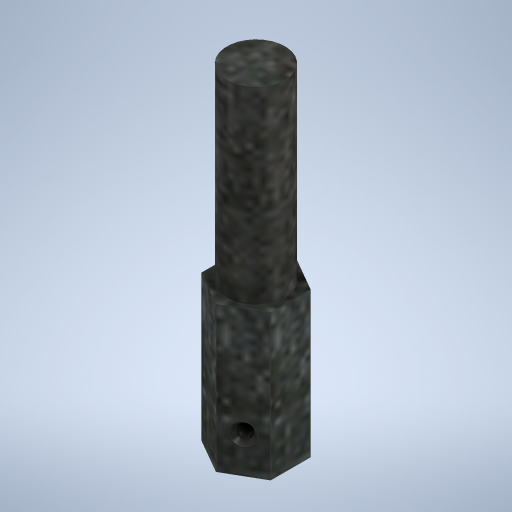
# Autodesk Inventor part: bevel gear shaft connector for versaball
Saved by Autodesk Inventor 2023 (Build 270158030, 158C)
## iProperties
Created: 2022-10-20
Part Number: bevel gear shaft connector for versaball
Material: Steel
Document SubType Name: Modeling
Designer: cjj5381
Density: 7.85 g/cm^3
Appearance: Plate
Author: cjj5381
Autodesk Inventor part; units mm, degrees
ref_plane "YZ Plane" through (0, 0, 0) normal (1, 0, 0) x (0, 1, 0)
ref_plane "XZ Plane" through (0, 0, 0) normal (0, 1, 0) x (-1, 0, 0)
ref_plane "XY Plane" through (0, 0, 0) normal (0, 0, 1) x (1, 0, 0)
sketch "Sketch1" plane through (0, 0, 0) normal (0, 1, 0) x (-1, 0, 0)
  line L0 (0, -5.4993) -> (-4.7625, -2.7496)
  line L1 (-4.7625, -2.7496) -> (-4.7625, 2.7496)
  line L2 (-4.7625, 2.7496) -> (0, 5.4993)
  line L3 (0, 5.4993) -> (4.7625, 2.7496)
  line L4 (4.7625, 2.7496) -> (4.7625, -2.7496)
  line L5 (4.7625, -2.7496) -> (0, -5.4993)
  point P0 (0, 0)
  point P1 (0, 0)
  dimension "d0" = 9.525
  constraints: 12 end point, 1 coincident, 13 other
  measures "d0" distance between parallel lines of L1 L4
extrude "Extrusion1" add sketch "Sketch1" along normal blind 20
sketch "Sketch2" plane through (0, 20, 0) normal (0, 1, 0) x (1, 0, 0)
  circle A0 centre (0, 0) radius 4
  dimension "d3" = 8
  constraints: 1 centre point, 1 coincident
  measures "d3" diameter of A0
extrude "Extrusion2" add sketch "Sketch2" along normal blind 5
sketch "Sketch4" plane through (4.7625, 0, 2.7496) normal (0.5, 0, 0.8660254) x (0.8660254, 0, -0.5)
  line L0 (-5.4993, 0) -> (0, 0) projected
  line L1 (0, 0) -> (0, 20) projected
  point P0 (-2.7496, 0)
  point P1 (-2.75, 5)
  dimension "d13" = 5
  dimension "d21" = 2.75
  measures "d13" distance from line of L0 point (-2.75, 5)
  measures "d21" distance from line of L1 point (-2.75, 5)
hole "Hole1" at (2.3809, 5, 4.1246) direction (-0.5, 0, -0.8660254) diameter 2 end through all countersink diameter 3 countersink angle 82
sketch "Sketch5" plane through (0, 25, 0) normal (0, 1, 0) x (1, 0, 0)
  circle A0 centre (0, 0) radius 4 projected
  circle A1 centre (0, 0) radius 4
  constraints: 1 centre point, 1 coincident
extrude "Extrusion4" add sketch "Sketch5" along normal blind 21
body "Solid1"
